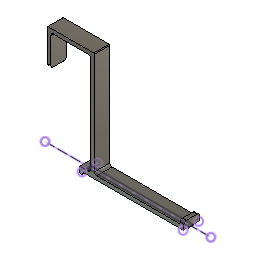
POT-HANGER (Autodesk Fusion 360 design; units mm, degrees)
Autodesk Fusion 360 part; units mm, degrees
note: some values were not read from the file. Chosen so that the rebuilt part matches the saved one: which face or edge a step refers to. Set by a fixed rule: which sketch regions a step uses.
sketch "Sketch1" plane through (0, 0, 0) normal (0, 1, 0) x (1, 0, 0)
  line L0 (0, 0) -> (0, -5)
  line L1 (0, -5) -> (14, -5)
  line L2 (14, -5) -> (14, -136)
  line L3 (14, -136) -> (-37.5, -136)
  line L4 (-37.5, -136) -> (-37.5, -96)
  line L5 (-37.5, -96) -> (-42.5, -96)
  line L6 (-42.5, -96) -> (-42.5, -141)
  line L7 (-42.5, -141) -> (19, -141)
  line L8 (19, -141) -> (19, -5)
  line L9 (19, -5) -> (130, -5)
  line L10 (130, -5) -> (130, -10)
  line L11 (130, -10) -> (135, -10)
  line L12 (135, -10) -> (135, 0)
  line L13 (135, 0) -> (0, 0)
  dimension "d1" = 5
  dimension "d2" = 51.5
  dimension "d3" = 5
  dimension "d4" = 5
  dimension "d5" = 5
  dimension "d6" = 5
  dimension "d7" = 5
  dimension "d8" = 14
  dimension "d9" = 130
  dimension "d10" = 5
  dimension "d11" = 131
  dimension "d12" = 40
  constraint coincident L0.start L13.end
  constraint vertical L0
  constraint perpendicular L0 L1
  constraint perpendicular L1 L2
  constraint perpendicular L2 L3
  constraint perpendicular L3 L4
  constraint perpendicular L4 L5
  constraint perpendicular L3 L6
  constraint perpendicular L6 L7
  constraint perpendicular L7 L8
  constraint perpendicular L8 L9
  constraint perpendicular L9 L10
  constraint perpendicular L10 L11
  constraint perpendicular L11 L12
  constraint perpendicular L0 L13
  measures "d1" distance of L4.end L5.end
  measures "d2" distance of L2.end L3.end
  measures "d3" distance of L3 L7
  measures "d4" distance of L2 L8
  measures "d5" distance of L10.end L11.end
  measures "d6" distance of L0.start L0.end
  measures "d7" distance of L9 L13
  measures "d8" distance of L0 L2
  measures "d9" distance of L0 L10
  measures "d10" distance of L9 L11
  measures "d11" distance of L3 L9
  measures "d12" distance of L3 L5.end
extrude "Extrude1" add sketch "Sketch1" along normal blind 20
fillet "Fillet1" radius 3 1 edges at (-37.5, 10, 136)
fillet "Fillet2" radius 3 1 edges at (14, 10, 136)
fillet "Fillet3" radius 3 1 edges at (14, 10, 5)
fillet "Fillet4" radius 3 1 edges at (19, 10, 5)
fillet "Fillet5" radius 1 1 edges at (130, 10, 5)
fillet "Fillet6" radius 1 1 edges at (135, 10, 0)
fillet "Fillet7" radius 3 2 edges at (132.5, 0, 10) (132.5, 20, 10)
fillet "Fillet9" radius 1 1 edges at (-42.5, 10, 141)
fillet "Fillet10" radius 3 2 edges at (-40, 0, 96) (-40, 20, 96)
fillet "Fillet11" radius 1 1 edges at (19, 10, 141)
sketch "Sketch2" plane through (0, 0, 0) normal (-1, 0, 0) x (0, -1, 0)
  line L0 (0, 0) -> (0, 5)
  line L1 (0, 5) -> (-20, 5)
  line L2 (-20, 5) -> (-20, 0)
  line L3 (-20, 0) -> (0, 0)
  line L4 (-20, 4.5) -> (0, 4.5)
  line L5 (0, 4.5) -> (0, -3)
  line L6 (0, -3) -> (-20, -3)
  line L7 (-20, -3) -> (-20, 4.5)
  dimension "d48" = 3
  constraint horizontal L4
  constraint vertical L5
  constraint horizontal L6
  constraint vertical L7
  measures "d48" distance of L3 L6
extrude "Extrude2" add sketch "Sketch2" against normal blind 3 contours L0 L2 L3 L4 L5 L7 | L3 L5 L6 L7
fillet "Fillet12" radius 3 1 edges at (3, 10, 0)
sketch "Sketch3" plane through (0, 0, 0) normal (0, 0, -1) x (1, 0, 0)
  line L0 (6, 0) -> (6, -20)
  line L1 (6, -20) -> (134, -20)
  line L2 (134, -20) -> (134, 0)
  line L3 (134, 0) -> (6, 0)
  line L4 (-55, -10) -> (160, -10) construction
  dimension "d41" = 10
  constraint parallel L3 L4
  measures "d41" distance of origin L4
sketch "Sketch4" plane through (0, 0, 0) normal (0, 0, -1) x (1, 0, 0)
  line L0 (3, -10) -> (3, -7.5)
  line L1 (3, -7.5) -> (134, -7.5)
  line L2 (134, -7.5) -> (134, -12.5)
  line L3 (134, -12.5) -> (3, -12.5)
  line L4 (3, -12.5) -> (3, -10)
  line L5 (-55, -10) -> (160, -10)
  line L6 (134, -20) -> (134, 0)
  line L7 (3, 0) -> (3, -20)
  dimension "d42" = 2.5
  dimension "d43" = 2.5
  constraint vertical L0
  constraint perpendicular L0 L1
  constraint perpendicular L1 L2
  constraint perpendicular L0 L3
  constraint perpendicular L3 L4
  constraint collinear L2 L6
  constraint collinear L0 L7
  measures "d42" distance of L1 L5
  measures "d43" distance of L3 L5
extrude "Extrude3" add sketch "Sketch4" along normal blind 3
fillet "Fillet13" radius 1 2 edges at (3.8787, 7.5, -0.8787) (70, 7.5, 0)
fillet "Fillet14" radius 2 2 edges at (70, 12.5, 0) (3.8787, 12.5, -0.8787)
fillet "Fillet15" radius 3 1 edges at (134, 10, -3)
